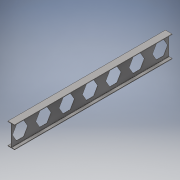
# Autodesk Inventor part: CastUB 1371x419x388
Saved by Autodesk Inventor 2021 (Build 250183000, 183)
## iProperties
Created: 2021-01-21
Part Number: CastUB 1371x419x388
Material: Steel, Mild
Document SubType Name: Modeling
Designer: David Brough
Density: 7.85 g/cm^3
Appearance: Semi-Polished
Author: David Brough
Autodesk Inventor part; units mm, degrees
note: some values were not read from the file. Chosen so that the rebuilt part matches the saved one: pattern direction of "Rectangular Pattern1".
ref_plane "YZ Plane" through (0, 0, 0) normal (1, 0, 0) x (0, 1, 0)
ref_plane "XZ Plane" through (0, 0, 0) normal (0, 1, 0) x (-1, 0, 0)
ref_plane "XY Plane" through (0, 0, 0) normal (0, 0, 1) x (1, 0, 0)
sketch "Sketch1" plane through (0, 0, 0) normal (0, 0, 1) x (1, 0, 0)
  line L0 (209.5, 689) -> (-209.5, 689)
  line L1 (-209.5, 689) -> (-209.5, 652.4)
  line L2 (-209.5, 652.4) -> (-34.8, 652.4)
  line L3 (-10.7, 628.3) -> (-10.7, -628.3)
  line L4 (-34.8, -652.4) -> (-209.5, -652.4)
  line L5 (-209.5, -652.4) -> (-209.5, -689)
  line L6 (-209.5, -689) -> (209.5, -689)
  line L7 (209.5, -689) -> (209.5, -652.4)
  line L8 (209.5, -652.4) -> (34.8, -652.4)
  line L9 (10.7, -628.3) -> (10.7, 628.3)
  line L10 (34.8, 652.4) -> (209.5, 652.4)
  line L11 (209.5, 652.4) -> (209.5, 689)
  arc A0 (-10.7, 628.3) -> (-34.8, 652.4) centre (-34.8, 628.3) ccw
  arc A1 (34.8, 652.4) -> (10.7, 628.3) centre (34.8, 628.3) ccw
  arc A2 (-34.8, -652.4) -> (-10.7, -628.3) centre (-34.8, -628.3) ccw
  arc A3 (10.7, -628.3) -> (34.8, -652.4) centre (34.8, -628.3) ccw
  line L12 (-10.7, 0) -> (10.7, 0) construction
  point P0 (0, 0)
  point P1 (0, 0)
  dimension "d0" = 1378
  dimension "d1" = 419
  dimension "d2" = 21.4
  dimension "d3" = 36.6
  dimension "d4" = 24.1
  constraints: 26 end point, 11 perpendicular, 8 point on circle, 8 tangent, 6 collinear, 4 centre point, 3 equal radius, 3 midpoint, 1 coincident, 1 horizontal
  measures "d0" distance between parallel lines of L6 L0
  measures "d1" distance of L0.start L0.end
  measures "d2" distance between parallel lines of L3 L9
  measures "d3" distance of L0.end L1.end
  measures "d4" radius of A0
extrude "Extrusion1" add sketch "Sketch1" against normal mid plane 10000
sketch "Sketch2" plane through (10.7, -628.3, -5000) normal (1, 0, 0) x (0, 0, -1)
  line L0 (-5229.7109, 1085.3) -> (-4770.2891, 1085.3)
  line L1 (-4770.2891, 171.3) -> (-5229.7109, 171.3)
  line L2 (-5229.7109, 1085.3) -> (-5493.56, 628.3)
  line L3 (-5493.56, 628.3) -> (-5229.7109, 171.3)
  line L4 (-4770.2891, 1085.3) -> (-4506.44, 628.3)
  line L5 (-4506.44, 628.3) -> (-4770.2891, 171.3)
  line L6 (0, 1317.3) -> (-10000, 1317.3) projected
  line L7 (-10000, 0) -> (-10000, 1256.6) projected
  point P0 (-5000, 628.3)
  point P1 (-5000, 1085.3)
  point P2 (-5000, 171.3)
  point P3 (-5000, 1317.3)
  point P4 (-10000, 628.3)
  dimension "d7" = 914
  dimension "d9" = 120
  dimension "d10" = 987.12
  constraints: 12 end point, 4 midpoint, 3 equal length, 3 horizontal alignment, 3 vertical alignment, 1 horizontal, 1 parallel
  measures "d7" distance between parallel lines of L1 L0
  measures "d9" angle of L3 L2
  measures "d10" distance of L4.end L2.end
extrude "Extrusion2" cut sketch "Sketch2" along normal through all both and the other way through all
pattern_linear "Rectangular Pattern1" count 4 spacing 1480.68 along (0, 0, 1) count 4 spacing 1480.68 along (0, 0, -1) of "Extrusion2"
equation "\"d0\" = cast_height"
equation "\"d1\" = original_width"
equation "\"d2\" = thk_web"
equation "\"d3\" = thk_flange"
equation "\"d4\" = root_rad"
equation "\"d5\" = beam_length"
equation "\"d7\" = cast_cutout_height"
equation "\"d10\" = cast_cutout_width"
equation "\"d13\" = 0.5 * cast_cutout_qty"
equation "\"d15\" = cast_cutout_spacing"
equation "\"d18\" = 0.5 * cast_cutout_qty"
equation "\"d20\" = cast_cutout_spacing"
equation "\"oiginal_height\" = 914"
equation "\"original_width\" = 419"
equation "\"thk_web\" = 21.4"
equation "\"thk_flange\" = 36.6"
equation "\"root_rad\" = 24.1"
equation "\"cast_height\" = 1378"
equation "\"cast_cutout_height\" = oiginal_height"
equation "\"cast_cutout_width\" = 1.08 * oiginal_height"
equation "\"cast_cutout_spacing\" = 1.5 * cast_cutout_width"
equation "\"beam_length\" = 10000"
equation "\"cast_end_cutout_offset\" = 0.5 * cast_cutout_spacing"
equation "\"cast_cutout_qty\" = 7"
body "Solid1"
